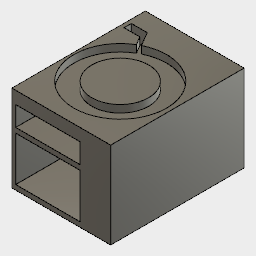
Pumpkin-Candle (Autodesk Fusion 360 design; units mm, degrees)
Autodesk Fusion 360 part; units mm, degrees
note: some values were not read from the file. Set by a fixed rule: which sketch regions a step uses.
sketch "Sketch1" plane through (0, 0, 0) normal (0, 1, 0) x (1, 0, 0)
  line L0 (-46.4072, 33.7716) -> (-20.4072, 33.7716)
  line L1 (-20.4072, 33.7716) -> (-20.4072, -17.2284)
  line L2 (-20.4072, -17.2284) -> (-46.4072, -17.2284)
  line L3 (-46.4072, -17.2284) -> (-46.4072, 33.7716)
  line L4 (-46.4072, -17.2284) -> (-28.4072, -17.2284)
  line L5 (-28.4072, -17.2284) -> (-28.4072, 27.7716)
  line L6 (-28.4072, 27.7716) -> (-46.4072, 27.7716)
  line L7 (-46.4072, 27.7716) -> (-46.4072, -17.2284)
  line L8 (-28.4072, -17.2284) -> (-12.9072, -17.2284)
  line L9 (-12.9072, -17.2284) -> (-12.9072, 11.7716)
  line L10 (-12.9072, 11.7716) -> (-28.4072, 11.7716)
  line L11 (-28.4072, 11.7716) -> (-28.4072, -17.2284)
  circle A0 centre (-28.4072, 5.2716) radius 18.75
  circle A1 centre (-28.4072, 5.2716) radius 11.5
  line L12 (-48, 35) -> (-48, -19)
  line L13 (-48, -19) -> (-8, -19)
  line L14 (-8, -19) -> (-8, 35)
  line L15 (-8, 35) -> (-48, 35)
  line L16 (-12.9072, -17.2284) -> (-8, -17.2284)
  line L17 (-46.4072, -17.2284) -> (-48, -17.2284)
  line L18 (-46.4072, -17.2284) -> (-46.4072, -19)
  line L19 (-20.4072, -17.2284) -> (-20.4072, -19)
  line L20 (-46.4072, 24.796) -> (-40, 24.796)
  line L21 (-40, 24.796) -> (-40, 27.7716)
  line L22 (-40, 24.796) -> (-37.9936, 21.3857)
  line L23 (-40, 27.7716) -> (-36.6659, 22.1048)
  dimension "d1" = 26
  dimension "d2" = 51
  dimension "d3" = 45
  dimension "d4" = 18
  dimension "d5" = 15.5
  dimension "d6" = 29
  dimension "d7" = 37.5
  dimension "d8" = 23
  measures "d1" distance of L0.start L0.end
  measures "d2" distance of L0.start L2.end
  measures "d3" distance of L2.end L6.end
  measures "d4" distance of L2.end L4.end
  measures "d5" distance of L4.end L8.end
  measures "d6" distance of L4.end L10.end
  measures "d7" diameter of A0
  measures "d8" diameter of A1
extrude "Extrude1" add sketch "Sketch1" along normal blind 2 makes body 1
extrude "Extrude2" add sketch "Sketch1" along normal blind 18 separate body contours L0 L1 L3 L7 L9 A0 L12 L14 L15 L16 L17 | L1 L9 L10 A0 A1 | L1 L10 A1 | L3 L7 A0 | L1 L10 A1 | L1 L9 L10 A0 A1 | L1 L8 L9 A0 | L8 L13 L14 L16 L19 | L12 L13 L17 L18 makes body 2
extrude "Extrude3" add sketch "Sketch1" along normal blind 2 separate body contours L0 L1 L3 L7 L9 A0 L12 L14 L15 L16 L17 | L0 L1 L3 L5 L6 A0 | L1 L9 L10 A0 A1 | L1 L5 A0 A1 | L3 L7 A0 L20 L22 | A0 L21 L22 L23 | L5 L6 A0 L23 | L1 L10 A1 | L1 L5 L10 A1 | L3 L5 L7 L11 A0 A1 | L3 L7 A0 | L1 L10 A1 | L1 L5 L10 L11 A1 | L1 L9 L10 A0 A1 | L5 L11 A1 | L1 L8 L9 A0 | L2 L3 L4 L5 L7 L11 A0 | L1 L5 L11 A0 A1 | L8 L13 L14 L16 L19 | L1 L2 L5 L8 L11 A0 | L12 L13 L17 L18 | L2 L4 L8 L13 L18 L19 makes body 3
extrude "Extrude4" add sketch "Sketch1" along normal blind 8 separate body contours L0 L1 L3 L7 L9 A0 L12 L14 L15 L16 L17 | L0 L1 L3 L5 L6 A0 | L1 L9 L10 A0 A1 | L1 L5 A0 A1 | L1 L10 A1 | L1 L5 L10 A1 | L3 L7 A0 | L8 L13 L14 L16 L19 | L12 L13 L17 L18 picked at (-14.7995, 12.9513) picked at (-19.8853, 12.3809) makes body 4
extrude "Extrude5" add sketch "Sketch1" along normal blind 2 separate body contours L0 L1 L3 L7 L9 A0 L12 L14 L15 L16 L17 | L0 L1 L3 L5 L6 A0 | L1 L9 L10 A0 A1 | L1 L5 A0 A1 | L3 L7 A0 L20 L22 | A0 L21 L22 L23 | L5 L6 A0 L23 | L1 L10 A1 | L1 L5 L10 A1 | L3 L5 L7 L11 A0 A1 | L3 L7 A0 | L1 L10 A1 | L1 L5 L10 L11 A1 | L1 L9 L10 A0 A1 | L5 L11 A1 | L1 L8 L9 A0 | L2 L3 L4 L5 L7 L11 A0 | L1 L5 L11 A0 A1 | L8 L13 L14 L16 L19 | L1 L2 L5 L8 L11 A0 | L12 L13 L17 L18 | L2 L4 L8 L13 L18 L19 makes body 5
extrude "Extrude6" add sketch "Sketch1" along normal blind 3 separate body contours L0 L1 L3 L7 L9 A0 L12 L14 L15 L16 L17 | L0 L1 L3 L5 L6 A0 | L3 L7 A0 L20 L22 | L5 L6 A0 L23 | L1 L10 A1 | L1 L5 L10 A1 | L1 L10 A1 | L1 L5 L10 L11 A1 | L5 L11 A1 | L1 L8 L9 A0 | L2 L3 L4 L5 L7 L11 A0 | L8 L13 L14 L16 L19 | L1 L2 L5 L8 L11 A0 | L12 L13 L17 L18 | L2 L4 L8 L13 L18 L19 makes body 6 at (-32, 3, -32.5905) makes body 7 at (-31.134, 0, -9.3605)
move_body "Move1" bodies 2 to x (1, 0, 0) y (0, 1, 0) z (0, 0, 1) at (0, 2, 0)
move_body "Move2" bodies 3 to x (1, 0, 0) y (0, 1, 0) z (0, 0, 1) at (0, 20, 0)
move_body "Move3" bodies 4 to x (1, 0, 0) y (0, 1, 0) z (0, 0, 1) at (0, 22, 0)
move_body "Move4" bodies 5 to x (1, 0, 0) y (0, 1, 0) z (0, 0, 1) at (0, 30, 0)
move_body "Move5" bodies 6 to x (1, 0, 0) y (0, 1, 0) z (0, 0, 1) at (0, 32, 0)
move_body "Move6" bodies 7 to x (1, 0, 0) y (0, 1, 0) z (0, 0, 1) at (0, 32, 0)
combine "Combine1" operation add target body 1 tool bodies 7 6 2 4 3 5
named bodies: "Base", "Battery Layer", "Battery Roof", "Board Layer", "Board Roof", "Roof", "Roof Ring Inset"
